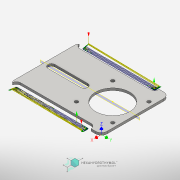
# Autodesk Inventor part: X-motor-holder
Saved by Autodesk Inventor 2016 (Build 200138000, 138)
## iProperties
Created: 2015-05-16
Part Number: X-motor-holder
Material: Generic
Document SubType Name: Modeling
Designer: as
Density: 1 g/cm^3
Appearance: Default
Mass: 6.59762 g
Surface Area: 75.7711 cm^2
Volume: 6.59762 cm^3
Author: as
Autodesk Inventor part; units mm, degrees
ref_plane "YZ Plane" through (0, 0, 0) normal (1, 0, 0) x (0, 1, 0)
ref_plane "XZ Plane" through (0, 0, 0) normal (0, 1, 0) x (-1, 0, 0)
ref_plane "XY Plane" through (0, 0, 0) normal (0, 0, 1) x (1, 0, 0)
sketch "Sketch1" plane through (0, 0, 0) normal (0, 0, 1) x (1, 0, 0)
  circle A0 centre (0, 0) radius 15 projected
  circle A1 centre (16, 16) radius 1.5 projected
  circle A2 centre (-16, 16) radius 1.5 projected
  circle A3 centre (-16, -16) radius 1.5 projected
  circle A4 centre (16, -16) radius 1.5 projected
  line L0 (20, -18) -> (20, 18) projected
  line L1 (18, 20) -> (-18, 20) projected
  line L2 (-60.0198, 26.9978) -> (-59.9853, -20.0189)
  line L3 (-18, -20) -> (18, -20) projected
  line L4 (-57.0198, 30) -> (-15.022, 30)
  line L5 (-14.978, -30) -> (-56.9802, -30)
  line L6 (-59.9802, -27.0022) -> (-60.0198, 26.9978)
  arc A5 (-59.9802, -27.0022) -> (-56.9802, -30) centre (-56.9802, -27) ccw
  arc A6 (-57.0198, 30) -> (-60.0198, 26.9978) centre (-57.0198, 27) ccw
  line L7 (20, -18) -> (20, 18)
  line L8 (-14.978, -30) -> (20, -30)
  line L9 (20, -30) -> (20, -18)
  line L10 (20, -30) -> (-56.9802, -30)
  line L11 (-60.0198, -29) -> (-60.0198, 27)
  line L12 (-57.0198, 30) -> (20, 30)
  line L13 (20, 30) -> (20, -30)
  point P0 (0, 0)
  point P1 (-60.0198, 26.9811)
  point P2 (-59.978, -30)
  dimension "d16" = 3
  dimension "d17" = 3
  dimension "d26" = 30
  dimension "d27" = 60
  dimension "d29" = 45
  dimension "d30" = 45
  dimension "d31" = 60
  dimension "d32" = 79.9853
  dimension "d33" = 80.0198
  constraints: 22 end point, 5 point on circle, 5 tangent, 4 point on line, 3 parallel, 3 perpendicular, 2 centre point, 2 horizontal, 1 vertical
  measures "d16" radius of A5
  measures "d17" radius of A6
  measures "d26" distance from line of point (0, 0) L5
  measures "d27" distance between parallel lines of L4 L5
  measures "d29" distance from line of L4.end L2
  measures "d30" distance from line of L2 L5.start
  measures "d31" distance from line of point (0, 0) L6
  measures "d32" distance from line of L2.end L0
  measures "d33" distance from line of point (-60.02, 26.981) L0
extrude "Extrusion1" add sketch "Sketch1" along normal blind 2
fillet "Fillet1" radius 5 2 edges at (20, -30, 1) (20, 30, 1)
sketch "Sketch4" plane through (0, 0, 2) normal (0, 0, 1) x (1, 0, 0)
  line L0 (-21.95, -0.0183) -> (-57.05, -0.0183) construction
  line L1 (-25, 3.0317) -> (-54, 3.0317)
  line L2 (-54, -3.0683) -> (-25, -3.0683)
  arc A0 (-25, -3.0683) -> (-25, 3.0317) centre (-25, -0.0183) ccw
  arc A1 (-54, 3.0317) -> (-54, -3.0683) centre (-54, -0.0183) ccw
  circle A2 centre (0, 0) radius 15 projected
  line L3 (-60.0198, 26.9978) -> (-59.9802, -27.0022) projected
  point P0 (0, 0)
  point P1 (-39.5, -0.0183)
  dimension "d34" = 6.1
  dimension "d35" = 25
  dimension "d36" = 6
  constraints: 8 end point, 6 point on circle, 4 tangent, 2 centre point, 2 point on line, 1 horizontal, 1 midpoint, 1 parallel
  measures "d34" diameter of A1
  measures "d35" distance of A2.centre A0.centre
  measures "d36" distance from line of L3 A1.centre
extrude "Extrusion2" cut sketch "Sketch4" against normal through all contours A0 L2 A1 L1
sketch "Sketch5" plane through (0, 0, 2) normal (0, 0, 1) x (1, 0, 0)
  point P0 (0, 0)
sketch "Sketch6" plane through (0, 0, 2) normal (0, 0, 1) x (1, 0, 0)
  line L0 (15, 30) -> (-57.0198, 30) projected
  line L1 (7, 30) -> (-55, 30) construction
  line L2 (7, 34) -> (-55, 34)
  line L3 (-55, 26) -> (7, 26)
  arc A0 (7, 26) -> (7, 34) centre (7, 30) ccw
  arc A1 (-55, 34) -> (-55, 26) centre (-55, 30) ccw
  point P0 (0, 0)
  point P1 (-24, 30)
  dimension "d39" = 62
  constraints: 8 end point, 4 point on circle, 4 tangent, 2 centre point, 2 point on line, 1 midpoint, 1 parallel
  measures "d39" distance of L3.start L3.end
extrude "Extrusion3" cut sketch "Sketch6" against normal through all
ref_plane "Work Plane1" through (15, 0, 2) normal (0, 1, 0) x (1, 0, 0)
mirror "Mirror1" about plane through (15, 0, 2) normal (0, 1, 0) of "Extrusion3"
equation "\"d26\" = 0.5 * d27"
equation "\"d30\" = d29"
body "Solid1"
